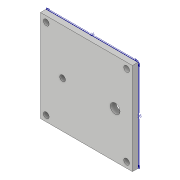
# Autodesk Inventor part: cappingsystem 3rd part
Saved by Autodesk Inventor 2019 (Build 230136000, 136)
## iProperties
Created: 2019-10-12
Part Number: cappingsystem 3rd part
Material: Generic
Document SubType Name: Modeling
Designer: Admin
Density: 1 g/cm^3
Appearance: Default
Author: Admin
Autodesk Inventor part; units mm, degrees
ref_plane "YZ Plane" through (0, 0, 0) normal (1, 0, 0) x (0, 1, 0)
ref_plane "XZ Plane" through (0, 0, 0) normal (0, 1, 0) x (-1, 0, 0)
ref_plane "XY Plane" through (0, 0, 0) normal (0, 0, 1) x (1, 0, 0)
sketch "Sketch1" plane through (0, 0, 0) normal (0, 0, 1) x (1, 0, 0)
  line L0 (0, 0) -> (160, 0)
  line L1 (160, 0) -> (160, 160)
  line L2 (160, 160) -> (0, 160)
  line L3 (0, 160) -> (0, 0)
  dimension "d0" = 160
  dimension "d1" = 160
  constraints: 8 end point, 2 parallel, 1 horizontal, 1 perpendicular
  measures "d0" distance of L2.end L1.end
  measures "d1" distance of L1.end L0.end
extrude "Extrusion1" add sketch "Sketch1" along normal blind 10
sketch "Sketch2" plane through (0, 0, 10) normal (0, 0, 1) x (1, 0, 0)
  line L0 (0, 160) -> (0, 0) projected
  line L1 (0, 0) -> (10, 0)
  line L2 (0, 0) -> (160, 0) projected
  line L3 (10, 0) -> (10, 150)
  line L4 (10, 150) -> (150, 150)
  line L5 (150, 150) -> (150, 10)
  line L6 (150, 10) -> (10, 10)
  line L7 (0, 0) -> (0, 10)
  line L8 (0, 0) -> (0, 2)
  line L9 (160, 160) -> (0, 160) projected
  line L10 (0, 160) -> (0, 121.5)
  line L11 (0, 160) -> (0, 80)
  line L12 (0, 80) -> (38.5, 80)
  circle A0 centre (38.5, 80) radius 5
  line L13 (160, 0) -> (160, 80)
  line L14 (160, 80) -> (130, 80)
  circle A1 centre (130, 80) radius 8.5
  dimension "d4" = 10
  dimension "d5" = 150
  dimension "d6" = 140
  dimension "d7" = 140
  dimension "d8" = 38.5
  dimension "d9" = 80
  dimension "d10" = 38.5
  dimension "d11" = 10
  dimension "d12" = 80
  dimension "d13" = 30
  dimension "d14" = 17
  constraints: 24 end point, 6 perpendicular, 5 point on line, 2 centre point, 2 coincident, 1 midpoint, 1 vertical
  measures "d4" distance of L0.end L1.end
  measures "d5" distance of L1.end L3.end
  measures "d6" distance of L3.end L4.end
  measures "d7" distance of L4.end L5.end
  measures "d8" distance of L0.start L10.end
  measures "d9" distance of L0.start L11.end
  measures "d10" distance of L11.end L12.end
  measures "d11" diameter of A0
  measures "d12" distance of L2.end L13.end
  measures "d13" distance of L13.end L14.end
  measures "d14" diameter of A1
sketch "Sketch3" plane through (0, 0, 10) normal (0, 0, 1) x (1, 0, 0)
  circle A0 centre (10, 10) radius 5
  circle A1 centre (10, 150) radius 5
  circle A2 centre (150, 150) radius 5
  circle A3 centre (150, 10) radius 5
  point P0 (0, 0)
  dimension "d15" = 10
  dimension "d16" = 10
  dimension "d17" = 10
  dimension "d18" = 10
  constraints: 4 centre point
  measures "d15" diameter of A0
  measures "d16" diameter of A1
  measures "d17" diameter of A2
  measures "d18" diameter of A3
extrude "Extrusion2" cut sketch "Sketch3" against normal through all
extrude "Extrusion3" cut sketch "Sketch2" against normal through all contours A1 | A0
body "Solid1"
